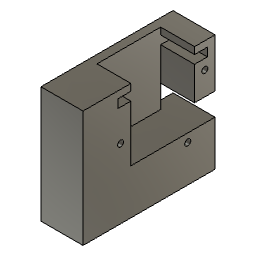
New Servo Mount Model v1 v1 (Autodesk Fusion 360 design; units mm, degrees)
Autodesk Fusion 360 part; units mm, degrees
sketch "Sketch1" plane through (0, 0, 0) normal (1, 0, 0) x (0, 1, 0)
  line L0 (-18.1754, 12.6139) -> (20.3246, 12.6139)
  line L1 (20.3246, 12.6139) -> (20.3246, -16.0861)
  line L2 (20.3246, -16.0861) -> (-18.1754, -16.0861)
  line L3 (-18.1754, -16.0861) -> (-18.1754, 12.6139)
  line L4 (20.3246, -10.1861) -> (12.7246, -10.1861)
  line L5 (12.7246, -10.1861) -> (12.7246, -1.8861)
  line L6 (12.7246, -1.8861) -> (20.3246, -1.8861)
  line L7 (20.3246, -1.8861) -> (20.3246, -10.1861)
  circle A0 centre (16.4746, 1.8639) radius 1.1
  circle A1 centre (-14.3254, -6.0861) radius 1.1
  dimension "d2" = 38.5
  dimension "d3" = 28.7
  dimension "d4" = 7.6
  dimension "d5" = 8.3
  dimension "d6" = 5.9
  dimension "d7" = 2.2
  dimension "d8" = 3.75
  dimension "d9" = 3.85
  dimension "d10" = 2.2
  dimension "d11" = 10
  dimension "d12" = 3.85
  constraint horizontal L0
  constraint vertical L1
  constraint horizontal L2
  constraint vertical L3
  constraint horizontal L4
  constraint vertical L5
  constraint horizontal L6
  constraint vertical L7
  constraint coincident L1 L4.start
  measures "d2" distance of L0.start L0.end
  measures "d3" distance of L0.start L2.end
  measures "d4" distance of L4.start L4.end
  measures "d5" distance of L4.start L6.end
  measures "d6" distance of L2 L4
  measures "d7" diameter of A0
  measures "d8" distance of L6 A0.centre
  measures "d9" distance of L1 A0.centre
  measures "d10" diameter of A1
  measures "d11" distance of L2 A1.centre
  measures "d12" distance of L3 A1.centre
extrude "Extrude1" add sketch "Sketch1" along normal blind 15.402 contours L0 L1 L2 L3 L4 L5 L6
sketch "Sketch2" plane through (15.402, 0, 0) normal (1, 0, 0) x (0, 1, 0)
  circle A0 centre (-14.3254, -6.0861) radius 1.1
  circle A1 centre (16.4746, 1.8639) radius 1.1
  line L0 (20.3246, -10.1861) -> (12.7246, -10.1861)
  line L1 (12.7246, -10.1861) -> (12.7246, -1.8861)
  line L2 (12.7246, -1.8861) -> (20.3246, -1.8861)
  line L3 (20.3246, -1.8861) -> (20.3246, 12.6139)
  line L4 (20.3246, 12.6139) -> (-18.1754, 12.6139)
  line L5 (-18.1754, 12.6139) -> (-18.1754, -16.0861)
  line L6 (-18.1754, -16.0861) -> (20.3246, -16.0861)
  line L7 (20.3246, -16.0861) -> (20.3246, -10.1861)
  line L8 (12.7246, -10.1861) -> (-10.5754, -10.1861)
  line L9 (-10.5754, -10.1861) -> (-10.5754, 12.6139)
  line L10 (-10.5754, 12.6139) -> (12.7246, 12.6139)
  line L11 (12.7246, 12.6139) -> (12.7246, -10.1861)
  line L12 (12.7246, 8.6139) -> (17.4246, 8.6139)
  line L13 (17.4246, 8.6139) -> (17.4246, 5.5139)
  line L14 (17.4246, 5.5139) -> (12.7246, 5.5139)
  line L15 (12.7246, 5.5139) -> (12.7246, 8.6139)
  line L16 (-10.5754, 5.5139) -> (-15.2754, 5.5139)
  line L17 (-15.2754, 5.5139) -> (-15.2754, 8.6139)
  line L18 (-15.2754, 8.6139) -> (-10.5754, 8.6139)
  line L19 (-10.5754, 8.6139) -> (-10.5754, 5.5139)
  dimension "d15" = 23.3
  dimension "d16" = 4.7
  dimension "d17" = 3.1
  dimension "d18" = 21.6
  dimension "d19" = 4.7
  dimension "d20" = 3.1
  dimension "d21" = 21.6
  constraint horizontal L8
  constraint vertical L9
  constraint horizontal L10
  constraint vertical L11
  constraint coincident L4 L9.end
  constraint coincident L0.end L1.start
  constraint horizontal L12
  constraint vertical L13
  constraint horizontal L14
  constraint vertical L15
  constraint coincident L11 L12.start
  constraint horizontal L16
  constraint vertical L17
  constraint horizontal L18
  constraint vertical L19
  constraint coincident L9 L16.start
  measures "d15" distance of L0.end L8.end
  measures "d16" distance of L12.start L12.end
  measures "d17" distance of L12.start L14.end
  measures "d18" distance of L6 L14
  measures "d19" distance of L17.end L18.end
  measures "d20" distance of L16.end L17.end
  measures "d21" distance of L6 L16
extrude "Extrude2" cut sketch "Sketch2" against normal blind 12.402 contours L1 L4 L8 L9 L10 L11 L15 L19 | L11 L12 L13 L14 L15 | L9 L16 L17 L18 L19
sketch "Sketch3" plane through (0, 0, 0) normal (-1, 0, 0) x (0, -1, 0)
  circle A0 centre (14.3254, -6.0861) radius 1.1
  circle A1 centre (-16.4746, 1.8639) radius 1.1
  line L0 (-12.7246, -10.1861) -> (-20.3246, -10.1861)
  line L1 (-20.3246, -10.1861) -> (-20.3246, -16.0861)
  line L2 (-20.3246, -16.0861) -> (18.1754, -16.0861)
  line L3 (18.1754, -16.0861) -> (18.1754, 12.6139)
  line L4 (18.1754, 12.6139) -> (-20.3246, 12.6139)
  line L5 (-20.3246, 12.6139) -> (-20.3246, -1.8861)
  line L6 (-20.3246, -1.8861) -> (-12.7246, -1.8861)
  line L7 (-12.7246, -1.8861) -> (-12.7246, -10.1861)
  circle A2 centre (-16.4746, 1.8639) radius 2.4
  circle A3 centre (14.3254, -6.0861) radius 2.4
  dimension "d24" = 4.8
  dimension "d25" = 4.8
  constraint concentric A1 A2
  constraint concentric A0 A3
  measures "d24" diameter of A2
  measures "d25" diameter of A3
extrude "Extrude3" cut sketch "Sketch3" against normal blind 7.701 contours A2
extrude "Extrude4" cut sketch "Sketch3" against normal blind 7.701 contours A3
extrude "Extrude5" cut 1 faces at (11.268, 7.4913, -10.1861) along direction (0, 0, -1) blind 4.8
extrude "Extrude6" add 1 faces at (5.134, 7.4913, -16.0861) along direction (0, 0, -1) blind 5
extrude "Extrude7" cut 1 faces at (5.134, 7.4913, -21.0861) along direction (0, 0, 1) blind 0.1
extrude "Extrude8" cut 1 faces at (5.134, -18.1754, 1.4139) along direction (0, 1, 0) blind 0.1
extrude "Extrude9" cut 1 faces at (5.134, 20.3246, 7.7806) along direction (0, -1, 0) blind 0.1
extrude "Extrude10" cut 1 faces at (5.134, 20.3246, -18.9861) along direction (0, -1, 0) blind 0.1
extrude "Extrude11" cut 1 faces at (6.134, 17.7246, 12.6139) along direction (0, 0, -1) blind 1
extrude "Extrude12" cut 1 faces at (6.134, 17.7246, 11.6139) along direction (0, 0, -1) blind 0.5
sketch "Sketch4" plane through (15.402, 0, 0) normal (1, 0, 0) x (0, 1, 0)
  line L0 (-10.5754, 11.1139) -> (-18.0754, 11.1139)
  line L1 (-18.0754, 11.1139) -> (-18.0754, -20.9861)
  line L2 (-18.0754, -20.9861) -> (20.2246, -20.9861)
  line L3 (20.2246, -20.9861) -> (20.2246, -14.9861)
  line L4 (20.2246, -14.9861) -> (-10.5754, -14.9861)
  line L5 (-10.5754, -14.9861) -> (-10.5754, 5.5139)
  line L6 (-10.5754, 5.5139) -> (-15.2754, 5.5139)
  line L7 (-15.2754, 5.5139) -> (-15.2754, 8.6139)
  line L8 (-15.2754, 8.6139) -> (-10.5754, 8.6139)
  line L9 (-10.5754, 8.6139) -> (-10.5754, 11.1139)
  circle A0 centre (-14.3254, -6.0861) radius 1.1
  circle A1 centre (10.2246, -18) radius 1.1
  dimension "d46" = 2.2
  dimension "d72" = 10
  measures "d46" diameter of A1
  measures "d72" distance of L3 A1.centre
extrude "Extrude13" cut sketch "Sketch4" against normal blind 15.402 contours A1
sketch "Sketch5" plane through (0, 0, 0) normal (-1, 0, 0) x (0, -1, 0)
  circle A0 centre (-10.2246, -18) radius 1.1
  line L0 (18.0754, 11.1139) -> (-20.2246, 11.1139)
  line L1 (-20.2246, 11.1139) -> (-20.2246, -1.8861)
  line L2 (-20.2246, -1.8861) -> (-12.7246, -1.8861)
  line L3 (-12.7246, -1.8861) -> (-12.7246, -14.9861)
  line L4 (-12.7246, -14.9861) -> (-20.2246, -14.9861)
  line L5 (-20.2246, -14.9861) -> (-20.2246, -20.9861)
  line L6 (-20.2246, -20.9861) -> (18.0754, -20.9861)
  line L7 (18.0754, -20.9861) -> (18.0754, 11.1139)
  circle A1 centre (14.3254, -6.0861) radius 2.4
  circle A2 centre (-16.4746, 1.8639) radius 2.4
  circle A3 centre (-10.2246, -18) radius 2.4
  dimension "d49" = 4.8
  constraint concentric A0 A3
  measures "d49" diameter of A3
extrude "Extrude14" cut sketch "Sketch5" against normal blind 7.701 contours A3
extrude "Extrude15" add 1 faces at (6.134, 17.7246, -1.8861) along direction (0, 0, -1) blind 4.8
extrude "Extrude16" add 1 faces at (5.134, 7.4579, -20.9861) along direction (0, 0, -1) blind 0.5
extrude "Extrude17" add 1 faces at (5.134, 7.4579, -21.4861) along direction (0, 0, -1) blind 10
extrude "Extrude18" add 1 faces at (5.134, -18.0754, -3.0861) along direction (0, -1, 0) blind 10
